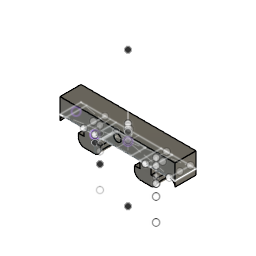
dimensionsTest (Autodesk Fusion 360 design; units mm, degrees)
part number: 2026-01-29-15-29-34-594
Autodesk Fusion 360 part; units mm, degrees
sketch "Sketch5" plane through (0, 0, 0) normal (0, 0, 1) x (1, 0, 0)
  line L0 (-41, -7.5) -> (41, -7.5)
  line L1 (41, -7.5) -> (41, 7.5)
  line L2 (41, 7.5) -> (-41, 7.5)
  line L3 (-41, 7.5) -> (-41, -7.5)
  line L4 (-41, -7.5) -> (41, 7.5) construction
  line L5 (41, -7.5) -> (-41, 7.5) construction
  line L6 (-37, 7.5) -> (-37, -7.5)
  line L7 (0, 7.5) -> (0, -7.5) construction
  line L8 (37, 7.5) -> (37, -7.5)
  line L9 (-10, -7.5) -> (10, -7.5) construction
  line L10 (10, -7.5) -> (10, 2.5)
  line L11 (10, 2.5) -> (-10, 2.5)
  line L12 (-10, 2.5) -> (-10, -7.5)
  line L13 (23.95, -7.5) -> (16.05, -7.5)
  line L14 (16.05, -7.5) -> (16.05, 7.5)
  line L15 (16.05, 7.5) -> (23.95, 7.5)
  line L16 (23.95, 7.5) -> (23.95, -7.5)
  line L17 (-23.95, 7.5) -> (-23.95, -7.5)
  line L18 (-16.05, -7.5) -> (-16.05, 7.5)
  line L19 (-20, -7.5) -> (-20, 7.5) construction
  line L20 (20, -7.5) -> (20, 7.5) construction
  dimension "d29" = 15
  dimension "d30" = 4
  dimension "d31" = 20
  dimension "d32" = 10
  dimension "d33" = 10
  dimension "d55" = 7.9
  dimension "d64" = 3.95
  dimension "d65" = 3.95
  dimension "d93" = 74
  dimension "d94" = 4
  dimension "d99" = 40
  constraint horizontal L0
  constraint perpendicular L0 L1
  constraint parallel L0 L2
  constraint parallel L1 L3
  constraint coincident L4 origin
  constraint coincident L5 origin
  constraint coincident L2 L6.start
  constraint coincident L0 L6.end
  constraint perpendicular L0 L6
  constraint midpoint L2 L7.start
  constraint midpoint L0 L7.end
  constraint symmetric L6.start L7 L8.start
  constraint symmetric L6.end L7 L8.end
  constraint horizontal L9
  constraint vertical L10
  constraint horizontal L11
  constraint vertical L12
  constraint coincident L0 L9.start
  constraint horizontal L13
  constraint vertical L14
  constraint horizontal L15
  constraint vertical L16
  constraint coincident L0 L13.start
  constraint symmetric L7 L13.start L17.end
  constraint symmetric L7 L13.end L18.start
  constraint symmetric L7 L14.end L18.end
  constraint symmetric L7 L15.end L17.start
  constraint coincident L0 L19.start
  constraint coincident L2 L19.end
  constraint perpendicular L2 L19
  constraint symmetric L7 L19.start L20.start
  constraint symmetric L7 L19.end L20.end
  constraint coincident L2 L18.end
  measures "d29" distance of L0.end L1.end
  measures "d30" distance of L3 L6
  measures "d31" distance of L10 L12
  measures "d32" distance of L7 L12
  measures "d33" distance of L9.start L11.end
  measures "d55" distance of L13.start L13.end
  measures "d64" distance of L17 L19
  measures "d65" distance of L18 L19
  measures "d93" distance of L6 L8
  measures "d94" distance of L1 L8
  measures "d99" distance of L19 L20
sketch "Sketch6" plane through (0, 0, 0) normal (0, 1, 0) x (1, 0, 0)
  circle A0 centre (0, -6) radius 2.6
  line L0 (0, -56.6756) -> (0, 40) construction
  line L1 (-20, 40) -> (-20, 0) construction
  line L2 (20, 40) -> (20, 0) construction
  line L3 (20, 40) -> (20, 0) construction
  line L4 (-1.3, -8.2517) -> (0, -9.0022)
  line L5 (-1.3, -8.2517) -> (0.2948, -8.2517) construction
  line L6 (1.3, -8.2517) -> (0, -9.0022)
  point P0 (0, -6)
  point P1 (0, -11)
  point P2 (0, -1)
  point P3 (0, -56.6756)
  point P4 (0, 40)
  point P5 (-20, 16)
  point P6 (20, 16)
  point P7 (-20, 12)
  point P8 (-20, 5)
  point P9 (20, 16)
  point P10 (20, 5)
  point P11 (-20, 24)
  point P12 (20, 24)
  point P13 (-24.75, 0)
  point P14 (-37, 0)
  point P15 (20, 24)
  point P16 (20, 12)
  point P17 (37, 0)
  point P18 (20, 16)
  point P19 (24.75, 0)
  point P20 (20, 5)
  dimension "d35" = 5.2
  dimension "d36" = 40
  dimension "d45" = 20
  dimension "d46" = 20
  dimension "d48" = 40
  dimension "d49" = 12
  dimension "d50" = 5
  dimension "d51" = 16
  dimension "d52" = 8
  dimension "d53" = 16
  dimension "d54" = 12.25
  dimension "d76" = 10
  dimension "d77" = 5
  dimension "d78" = 1
  dimension "d79" = 30
  constraint vertical P1 P3
  constraint vertical P0 P1
  constraint vertical P0 P2
  constraint vertical P2 origin
  constraint coincident P0 A0.centre
  constraint coincident P3 L0.start
  constraint coincident P4 L0.end
  constraint vertical L0
  constraint horizontal P5 P18
  constraint horizontal P4 L1.start
  constraint vertical P5 L1.start
  constraint coincident L1 P7
  constraint coincident L1 P8
  constraint symmetric P5 L0 P18
  constraint symmetric L0 L1.start L2.start
  constraint symmetric L0 L1.end L2.end
  constraint symmetric L0 P8 P20
  constraint coincident L1 P11
  constraint symmetric L0 P11 P15
  constraint symmetric L0 P7 P16
  constraint symmetric L0 P13 P19
  constraint symmetric L0 P14 P17
  constraint horizontal L5
  constraint coincident A0 L4.start
  constraint tangent A0 L4
  constraint symmetric L0 L4.start L6.start
  constraint symmetric L0 L4.end L6.end
  constraint coincident L0 L4.end
  measures "d35" diameter of A0
  measures "d36" distance of P4 origin
  measures "d45" distance of P5 L0
  measures "d46" distance of P18 L0
  measures "d48" distance of L1.start L1.end
  measures "d49" distance of L1.end P7
  measures "d50" distance of L1.end P8
  measures "d51" distance of P5 L1.end
  measures "d52" distance of P5 P11
  measures "d53" distance of L1.start P11
  measures "d54" distance of P13 P14
  measures "d76" distance of P1 P2
  measures "d77" distance of P0 P1
  measures "d78" distance of P2 origin
  measures "d79" angle of L4 L5
extrude "Extrude10" add sketch "Sketch5" along normal up to surface (11 mm away) makes body 1
extrude "Extrude14" add sketch "Sketch5" against normal up to surface (12 mm away) contours L0 L2 L17 L18 bodies 1
sketch "Sketch8" plane through (-16.05, 0, 0) normal (1, 0, 0) x (0, 1, 0)
  line L0 (-7.5, -12) -> (7.5, -12)
  line L1 (7.5, -12) -> (7.5, 0)
  line L2 (7.5, 0) -> (-7.5, 0)
  line L3 (-7.5, 0) -> (-7.5, -12)
  line L4 (-7.5, -5) -> (7.5, -5)
  line L5 (7.5, -5) -> (-7.5, -5)
  point P0 (-7.5, 0)
  dimension "d59" = 5
  constraint coincident L3 L4.start
  constraint coincident L1 L4.end
  constraint perpendicular L1 L4
  measures "d59" distance of L4.start P0
extrude "Extrude15" add sketch "Sketch8" along normal blind 4 contours L0 L1 L3 L4 L5 bodies 1
fillet "Fillet1" radius 4 tangency weight 0.7 1 edges at (-12.05, 0, -12) on bodies 1
sketch "Sketch9" plane through (-23.95, 0, 0) normal (-1, 0, 0) x (0, -1, 0)
  line L0 (-7.5, -12) -> (7.5, -12)
  line L1 (7.5, -12) -> (7.5, 0)
  line L2 (7.5, 0) -> (-7.5, 0)
  line L3 (-7.5, 0) -> (-7.5, -12)
  line L4 (-7.5, -5) -> (7.5, -5)
  line L5 (-7.5, 0) -> (7.5, 0)
  dimension "d67" = 5
  constraint coincident L3 L4.start
  constraint coincident L1 L4.end
  constraint perpendicular L1 L4
  measures "d67" distance of L4 L5
extrude "Extrude16" add sketch "Sketch9" along normal blind 4 contours L0 L1 L3 L4 bodies 1
fillet "Fillet2" radius 4 tangency weight 0.7 1 edges at (-27.95, 0, -12) on bodies 1
split "Split1" by plane through (0, 0, 0) normal (0, 0, 1) bodies 1 makes body 2 at (13.6667, -2.5, 11)
mirror "Mirror1" about plane through (0, 0, 0) normal (1, 0, 0) of bodies 1 makes body 3
extrude "Extrude17" cut sketch "Sketch6" along normal up to surface (15 mm away) from surface at -7.5 contours A0 bodies 2
extrude "Extrude18" add sketch "Sketch5" against normal blind 4 contours L0 L2 L3 L6 bodies 2
pipe "Pipe1" cut diameter 8 along 1 edges at (-37, 0, -4) on bodies 2 bodies 2
extrude "Extrude19" add sketch "Sketch5" against normal blind 4 contours L0 L1 L2 L8 bodies 2
pipe "Pipe2" cut diameter 8 along 1 edges at (37, 0, -4) on bodies 2 bodies 2
equation "d32 = d31 / 2"
equation "d46 = d45"
equation "d47 = 8 mm"
equation "d51 = d48 / 2 - d47 / 2"
equation "d59 = d50"
equation "d67 = d50"
equation "d77 = d76 / 2"
